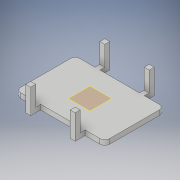
# Autodesk Inventor part: Floor
Saved by Autodesk Inventor 2019 (Build 230136000, 136)
## iProperties
Created: 2018-06-11
Part Number: Floor
Material: Ogólny
Document SubType Name: Modeling
Designer: Kamil
Density: 1 g/cm^3
Appearance: Domyślna
Author: Kamil
Autodesk Inventor part; units mm, degrees
ref_plane "YZ Plane" through (0, 0, 0) normal (1, 0, 0) x (0, 1, 0)
ref_plane "XZ Plane" through (0, 0, 0) normal (0, 1, 0) x (-1, 0, 0)
ref_plane "XY Plane" through (0, 0, 0) normal (0, 0, 1) x (1, 0, 0)
sketch "Szkic1" plane through (0, 0, 0) normal (0, 1, 0) x (-1, 0, 0)
  line L0 (40, -30) -> (25, -30)
  line L1 (-45, -25) -> (-45, 25)
  line L2 (-40, 30) -> (-25, 30)
  line L3 (45, 25) -> (45, -25)
  arc A0 (45, 25) -> (40, 30) centre (40, 25) ccw
  arc A1 (40, -30) -> (45, -25) centre (40, -25) ccw
  arc A2 (-45, -25) -> (-40, -30) centre (-40, -25) ccw
  arc A3 (-40, 30) -> (-45, 25) centre (-40, 25) ccw
  line L4 (40, 30) -> (35, 30)
  line L5 (20, 30) -> (20, 25)
  line L6 (20, 25) -> (25, 25)
  line L7 (25, 25) -> (25, 30)
  line L8 (2.5, 30) -> (-2.5, 30)
  line L9 (-25, 30) -> (-25, 25)
  line L10 (-25, 25) -> (-20, 25)
  line L11 (-20, 25) -> (-20, 30)
  line L12 (-35, 30) -> (-40, 30)
  line L13 (35, -30) -> (40, -30)
  line L14 (25, -25) -> (20, -25)
  line L15 (20, -25) -> (20, -30)
  line L16 (25, -30) -> (25, -25)
  line L17 (-2.5, -30) -> (2.5, -30)
  line L18 (-20, -25) -> (-25, -25)
  line L19 (-25, -25) -> (-25, -30)
  line L20 (-20, -30) -> (-20, -25)
  line L21 (-40, -30) -> (-35, -30)
  line L22 (20, -30) -> (-20, -30)
  line L23 (-25, -30) -> (-40, -30)
  line L24 (-20, 30) -> (20, 30)
  line L25 (25, 30) -> (40, 30)
  point P0 (0, 0)
  point P1 (40, -30)
  dimension "d2" = 5
  dimension "d5" = 5
  dimension "d6" = 5
  dimension "d9" = 5
  dimension "d12" = 5
  dimension "d13" = 5
  dimension "d15" = 5
  dimension "d17" = 5
  dimension "d19" = 5
  dimension "d21" = 5
  constraints: 52 end point, 16 tangent, 14 parallel, 8 horizontal, 8 point on circle, 5 perpendicular, 4 centre point, 3 equal radius, 3 point on line
  measures "d2" radius of A0
  measures "d5" distance of L6.end L5.end
  measures "d6" distance of L5.end L5.start
  measures "d9" distance of L10.end L9.end
  measures "d12" distance of A3.centre L12.end
  measures "d13" distance of L13.end L13.start
  measures "d15" distance of L0.end L15.end
  measures "d17" distance of L17.end L17.start
  measures "d19" distance of L20.start L19.end
  measures "d21" distance of L21.end L21.start
ref_plane "Płaszczyzna konstrukcyjna2" through (0, 0, 0) normal (0, -1, 0) x (1, 0, 0)
sketch "Szkic5" plane through (0, 0, 0) normal (0, -1, 0) x (1, 0, 0)
  line L0 (25, 25) -> (20, 25)
  line L1 (20, 25) -> (20, 40)
  line L2 (20, 40) -> (25, 40)
  line L3 (25, 40) -> (25, 25)
  line L4 (-20, 25) -> (-25, 25)
  line L5 (-25, 25) -> (-25, 40)
  line L6 (-25, 40) -> (-20, 40)
  line L7 (-20, 40) -> (-20, 25)
  line L8 (25, -25) -> (20, -25)
  line L9 (20, -25) -> (20, -40)
  line L10 (20, -40) -> (25, -40)
  line L11 (25, -40) -> (25, -25)
  line L12 (-20, -25) -> (-25, -25)
  line L13 (-25, -25) -> (-25, -40)
  line L14 (-25, -40) -> (-20, -40)
  line L15 (-20, -40) -> (-20, -25)
  point P0 (0, 0)
  dimension "d56" = 5
  dimension "d57" = 15
  dimension "d58" = 5
  dimension "d59" = 15
  dimension "d60" = 5
  dimension "d61" = 15
  dimension "d62" = 5
  dimension "d63" = 15
  constraints: 32 end point, 8 parallel, 4 horizontal, 4 perpendicular, 4 point on line
  measures "d56" distance of L1.end L2.end
  measures "d57" distance of L0.end L1.end
  measures "d58" distance of L5.end L6.end
  measures "d59" distance of L4.end L5.end
  measures "d60" distance of L10.end L9.end
  measures "d61" distance of L9.end L8.end
  measures "d62" distance of L14.end L13.end
  measures "d63" distance of L13.end L12.end
extrude "Wyciągnięcie proste5" add sketch "Szkic5" against normal blind 5
ref_plane "Płaszczyzna konstrukcyjna3" through (0, 5, 0) normal (0, 1, 0) x (1, 0, 0)
sketch "Szkic6" plane through (0, 5, 0) normal (0, 1, 0) x (1, 0, 0)
  line L0 (25, -40) -> (20, -40)
  line L1 (20, -40) -> (20, -35)
  line L2 (20, -35) -> (25, -35)
  line L3 (25, -35) -> (25, -40)
  line L4 (-20, -40) -> (-25, -40)
  line L5 (-25, -40) -> (-25, -35)
  line L6 (-25, -35) -> (-20, -35)
  line L7 (-20, -35) -> (-20, -40)
  line L8 (25, 40) -> (20, 40)
  line L9 (20, 40) -> (20, 35)
  line L10 (20, 35) -> (25, 35)
  line L11 (25, 35) -> (25, 40)
  line L12 (-20, 40) -> (-25, 40)
  line L13 (-25, 40) -> (-25, 35)
  line L14 (-25, 35) -> (-20, 35)
  line L15 (-20, 35) -> (-20, 40)
  point P0 (0, 0)
  dimension "d64" = 5
  dimension "d66" = 5
  dimension "d67" = 5
  dimension "d68" = 5
  dimension "d69" = 5
  dimension "d70" = 5
  dimension "d71" = 5
  dimension "d72" = 5
  dimension "d73" = 5
  constraints: 32 end point, 8 parallel, 4 horizontal, 4 perpendicular, 2 point on line
  measures "d66" distance of L1.end L2.end
  measures "d67" distance of L0.end L1.end
  measures "d68" distance of L5.end L6.end
  measures "d69" distance of L4.end L5.end
  measures "d70" distance of L10.end L9.end
  measures "d71" distance of L9.end L8.end
  measures "d72" distance of L14.end L13.end
  measures "d73" distance of L13.end L12.end
extrude "Wyciągnięcie proste6" add sketch "Szkic6" along normal blind 20
extrude "Wyciągnięcie proste7" add sketch "Szkic1" along normal blind 5
sketch "Szkic7" plane through (0, 0, 0) normal (0, -1, 0) x (1, 0, 0)
  point P0 (0, 0)
